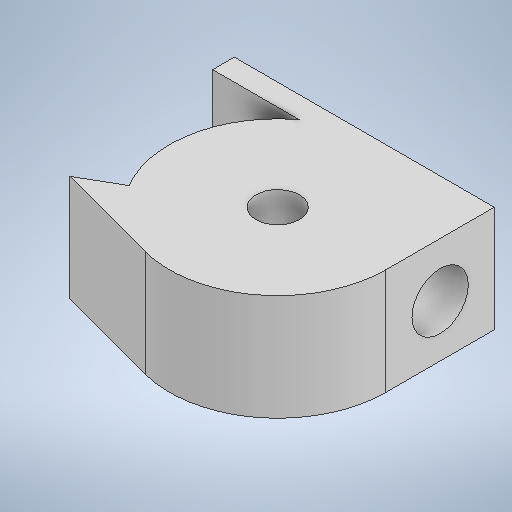
# Autodesk Inventor part: ikatire2b
Saved by Autodesk Inventor 2025 (Build 290162000, 162)
## iProperties
Created: 2024-04-11
Part Number: ikatire2b
Material: 一般
Document SubType Name: Modeling
Designer: Akio
Density: 1 g/cm^3
Appearance: 既定
Author: Akio
Autodesk Inventor part; units mm, degrees
ref_plane "YZ Plane" through (0, 0, 0) normal (1, 0, 0) x (0, 1, 0)
ref_plane "XZ Plane" through (0, 0, 0) normal (0, 1, 0) x (-1, 0, 0)
ref_plane "XY Plane" through (0, 0, 0) normal (0, 0, 1) x (1, 0, 0)
sketch "スケッチ1" plane through (0, 0, 0) normal (0, 1, 0) x (-1, 0, 0)
  arc A0 (0, -5) -> (-5, 0) centre (0, 0) ccw
  line L0 (0, -5) -> (-5, -5)
  line L1 (0, -5) -> (5, -5) construction
  line L2 (-5, -5) -> (-5, 0)
  dimension "d1" = 5
  dimension "d2" = 5
  dimension "d3" = 180
  dimension "d4" = 5
  constraints: 6 end point, 3 point on circle, 2 horizontal, 1 centre point, 1 coincident, 1 collinear
  measures "d1" distance of L2.end point (0, 0)
  measures "d2" distance of L0.start L0.end
  measures "d3" angle of L0 L1
  measures "d4" distance of L0.end L2.end
extrude "押し出し1" add sketch "スケッチ1" along normal blind 4.9
sketch "スケッチ2" plane through (0, 4.9, 0) normal (0, 1, 0) x (1, 0, 0)
  arc A0 (0, 5) -> (5, 0) centre (0, 0) ccw projected
  line L0 (0.0716, -4.9995) -> (0.0716, -6.9995)
  line L1 (0.0716, -6.9995) -> (3.5355, -3.5355)
  line L2 (0.0716, -6.9995) -> (4.9704, -6.9995) construction
  line L3 (0.0716, -4.9995) -> (3.5355, -3.5355)
  line L4 (4.3655, -2.4378) -> (6.0975, -3.4378)
  line L5 (6.0975, -3.4378) -> (4.8296, 1.2941)
  line L6 (4.3655, -2.4378) -> (4.8296, 1.2941)
  line L7 (4.2939, 2.5617) -> (6.0259, 3.5617)
  line L8 (6.0259, 3.5617) -> (1.2941, 4.8296)
  line L9 (4.2939, 2.5617) -> (1.2941, 4.8296)
  line L10 (-0.0716, 4.9995) -> (-0.0716, 6.9995)
  line L11 (-0.0716, 6.9995) -> (-3.5355, 3.5355)
  line L12 (-0.0716, 4.9995) -> (-3.5355, 3.5355)
  line L13 (-4.3655, 2.4378) -> (-6.0975, 3.4378)
  line L14 (-6.0975, 3.4378) -> (-4.8296, -1.2941)
  line L15 (-4.3655, 2.4378) -> (-4.8296, -1.2941)
  line L16 (-4.2939, -2.5617) -> (-6.0259, -3.5617)
  line L17 (-6.0259, -3.5617) -> (-1.2941, -4.8296)
  line L18 (-4.2939, -2.5617) -> (-1.2941, -4.8296)
  dimension "d7" = 2
  dimension "d8" = 45
  dimension "d41" = 360
  constraints: 38 end point, 3 point on circle, 1 equal length, 1 horizontal, 1 tangent, 1 vertical, 43 other
  measures "d7" distance of L0.start L0.end
  measures "d8" angle of L2 L1
sketch "スケッチ3" plane through (0, 4.9, 0) normal (0, 1, 0) x (1, 0, 0)
  point P0 (0, 0)
  point P1 (0, 0)
  constraints: 1 coincident
hole "穴1" at (0, 4.9, 0) direction (0, -1, 0) diameter 2 end through all
sketch "スケッチ4" plane through (5, 0, 0) normal (1, 0, 0) x (0, 0, -1)
  line L0 (0, 4.9) -> (5, 4.9) projected
  line L1 (5, 0) -> (5, 4.9) projected
  point P0 (0, 0)
  point P1 (2.5, 2.4)
  dimension "d28" = 2.5
  dimension "d29" = 2.5
  measures "d28" distance from line of L0 point (2.5, 2.4)
  measures "d29" distance from line of L1 point (2.5, 2.4)
hole "穴2" at (5, 2.4, -2.5) direction (-1, 0, 0) diameter 2.6 depth 5
sketch "スケッチ5" plane through (0, 4.9, 0) normal (0, 1, 0) x (1, 0, 0)
  point P0 (0, 0)
sketch "スケッチ7" plane through (0, 4.9, 0) normal (0, 1, 0) x (1, 0, 0)
  arc A0 (0, 5) -> (5, 0) centre (0, 0) ccw projected
  line L0 (0, 5) -> (-7, 5)
  line L1 (-7, 5) -> (-7, 4)
  line L2 (-7, 4) -> (-3, 4)
  line L3 (-3, 4) -> (0, 5)
  point P0 (-4.936, 0.7977)
  dimension "d35" = 7
  dimension "d36" = 1
  constraints: 8 end point, 1 horizontal, 1 perpendicular, 1 point on circle, 1 tangent, 1 vertical
  measures "d35" distance of L0.start L0.end
  measures "d36" distance of L0.end L1.end
extrude "押し出し4" add sketch "スケッチ7" against normal blind 4.9 contours A0 L2 L1 L0
extrude "押し出し5" add sketch "スケッチ2" against normal blind 4.9 contours A0 L17 L16
equation "\"d37\" = atumi"
equation "\"atumi\" = 4.9"
